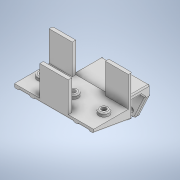
# Autodesk Inventor part: zMount1-2
Saved by Autodesk Inventor 2020 (Build 240168000, 168)
## iProperties
Created: 2020-01-08
Part Number: zMount1-2
Material: Generic
Document SubType Name: Modeling
Designer: PAB
Density: 1 g/cm^3
Appearance: Default
Author: PAB
Autodesk Inventor part; units mm, degrees
ref_plane "YZ Plane" through (0, 0, 0) normal (1, 0, 0) x (0, 1, 0)
ref_plane "XZ Plane" through (0, 0, 0) normal (0, 1, 0) x (-1, 0, 0)
ref_plane "XY Plane" through (0, 0, 0) normal (0, 0, 1) x (1, 0, 0)
sketch "Sketch1" plane through (0, 0, 0) normal (0, 1, 0) x (-1, 0, 0)
  line L0 (20.5, 16.2) -> (-20.5, 16.2)
  line L1 (-20.5, 16.2) -> (-20.5, -16.2)
  line L2 (-20.5, -16.2) -> (20.5, -16.2)
  line L3 (20.5, -16.2) -> (20.5, 16.2)
  point P0 (0, 0)
  dimension "d0" = 41
  dimension "d1" = 32.4
  constraints: 8 end point, 2 parallel, 1 horizontal, 1 perpendicular
  measures "d0" distance of L2.end L1.end
  measures "d1" distance of L1.end L0.end
extrude "Extrusion1" add sketch "Sketch1" along normal blind 3
sketch "Sketch3" plane through (0, 3, 0) normal (0, 1, 0) x (1, 0, 0)
  line L0 (-20.5, -16.2) -> (20.5, -16.2) projected
  line L1 (-20.5, 16.2) -> (-20.5, -16.2) projected
  line L2 (20.5, -16.2) -> (-20.5, -16.2)
  line L3 (-20.5, -16.2) -> (-20.5, -13.2)
  line L4 (-20.5, -13.2) -> (20.5, -13.2)
  line L5 (20.5, -13.2) -> (20.5, -16.2)
  line L6 (20.5, 16.2) -> (-20.5, 16.2) projected
  line L7 (20.5, 16.2) -> (-20.5, 16.2)
  line L8 (-20.5, 16.2) -> (-20.5, 13.2)
  line L9 (-20.5, 13.2) -> (20.5, 13.2)
  line L10 (20.5, 13.2) -> (20.5, 16.2)
  point P0 (0, 0)
  dimension "d8" = 3
  dimension "d9" = 3
  constraints: 16 end point, 4 parallel, 2 horizontal, 2 perpendicular, 2 point on line
  measures "d8" distance of L2.end L3.end
  measures "d9" distance of L8.end L7.end
extrude "Extrusion3" add sketch "Sketch3" along normal blind 25.4
sketch "Sketch4" plane through (20.5, 0, -16.2) normal (0, 0, -1) x (-1, 0, 0)
  line L0 (41, 3) -> (0, 3) projected
  line L1 (0, 28.4) -> (41, 28.4) projected
  line L2 (0, 3) -> (21.5, 3)
  line L3 (21.5, 3) -> (21.5, 28.4)
  line L4 (21.5, 28.4) -> (0, 28.4)
  line L5 (0, 28.4) -> (0, 3)
  point P0 (20.5, 0)
  dimension "d12" = 21.5
  constraints: 8 end point, 2 parallel, 1 horizontal, 1 perpendicular, 1 point on line
  measures "d12" distance of L4.end L3.end
extrude "Extrusion4" cut sketch "Sketch4" against normal blind 3
sketch "Sketch5" plane through (-20.5, 0, 16.2) normal (0, 0, 1) x (1, 0, 0)
  line L0 (41, 28.4) -> (0, 28.4) projected
  line L1 (19.5, 3) -> (41, 3) projected
  line L2 (0, 28.4) -> (21.5, 28.4)
  line L3 (21.5, 28.4) -> (21.5, 3)
  line L4 (21.5, 3) -> (0, 3)
  line L5 (0, 3) -> (0, 28.4)
  point P0 (20.5, 0)
  dimension "d15" = 21.5
  constraints: 8 end point, 2 parallel, 1 horizontal, 1 perpendicular, 1 point on line
  measures "d15" distance of L3.end L4.end
extrude "Extrusion5" cut sketch "Sketch5" against normal blind 3
sketch "Sketch6" plane through (0, 3, 0) normal (0, 1, 0) x (1, 0, 0)
  circle A0 centre (13, 0) radius 4.25
  circle A1 centre (-13, 0) radius 4.25
  line L0 (-20.5, 13.2) -> (-20.5, -16.2) projected
  line L1 (20.5, -13.2) -> (20.5, 16.2) projected
  point P0 (0, 0)
  dimension "d20" = 8.5
  dimension "d21" = 8.5
  dimension "d32" = 26
  dimension "d33" = 7.5
  dimension "d34" = 7.5
  constraints: 2 centre point
  measures "d20" diameter of A0
  measures "d21" diameter of A1
  measures "d32" distance of A0.centre A1.centre
  measures "d33" distance from line of L0 A1.centre
  measures "d34" distance from line of L1 A0.centre
extrude "Extrusion6" add sketch "Sketch6" along normal blind 3
sketch "Sketch9" plane through (20.5, 0, 16.2) normal (1, 0, 0) x (0, 0, -1)
  line L0 (32.4, 0) -> (32.4, 3) projected
  line L1 (32.4, 3) -> (0, 3)
  line L2 (0, 3) -> (0, 0)
  line L3 (0, 0) -> (32.4, 0)
  line L4 (32.4, 0) -> (32.4, 3)
  point P0 (16.2, 0)
  constraints: 8 end point, 2 parallel, 1 horizontal, 1 perpendicular
extrude "Extrusion9" add sketch "Sketch9" along normal blind 26
sketch "Sketch10" plane through (0, 3, 0) normal (0, 1, 0) x (1, 0, 0)
  circle A0 centre (39, 0) radius 4.25
  point P0 (0, 0)
  dimension "d37" = 8.5
  constraints: 1 centre point
  measures "d37" diameter of A0
extrude "Extrusion10" add sketch "Sketch10" along normal blind 3
sketch "Sketch11" plane through (0, 3, 0) normal (0, 1, 0) x (1, 0, 0)
  line L0 (46.5, 16.2) -> (46.5, -16.2) projected
  line L1 (46.5, 16.2) -> (27, 16.2)
  line L2 (27, 16.2) -> (27, 13.2)
  line L3 (27, 13.2) -> (46.5, 13.2)
  line L4 (46.5, 13.2) -> (46.5, 16.2)
  point P0 (0, 0)
  dimension "d40" = 19.5
  dimension "d41" = 3
  constraints: 8 end point, 2 parallel, 1 horizontal, 1 perpendicular
  measures "d40" distance of L3.end L2.end
  measures "d41" distance of L2.end L1.end
extrude "Extrusion11" add sketch "Sketch11" along normal blind 25.4
sketch "Sketch14" plane through (20.5, 3, 13.2) normal (1, 0, 0) x (0, 0, -1)
  line L0 (0, 0) -> (0, 25.4) projected
  line L1 (-3, 0) -> (-3, 25.4) projected
  line L2 (0, 25.4) -> (-3, 25.4)
  line L3 (-3, 25.4) -> (-3, 0)
  line L4 (-3, 0) -> (0, 0)
  line L5 (0, 0) -> (0, 25.4)
  point P0 (13.2, -3)
  constraints: 8 end point, 2 parallel, 1 horizontal, 1 perpendicular
extrude "Extrusion14" add sketch "Sketch14" along normal blind 4.5
fillet "Fillet1" radius 1 3 edges at (-17.25, 6, 0) (8.75, 6, 0) (34.75, 6, 0)
sketch "Sketch15" plane through (0, 0, 0) normal (0, -1, 0) x (1, 0, 0)
  circle A0 centre (39, 0) radius 4.25 projected
  circle A1 centre (39, 0) radius 2
  circle A2 centre (13, 0) radius 3.25 projected
  circle A3 centre (13, 0) radius 2
  circle A4 centre (-13, 0) radius 3.25 projected
  circle A5 centre (-13, 0) radius 2
  point P0 (0, 0)
  dimension "d54" = 4
  dimension "d55" = 4
  dimension "d56" = 4
  constraints: 3 centre point, 3 coincident
  measures "d54" diameter of A1
  measures "d55" diameter of A3
  measures "d56" diameter of A5
extrude "Extrusion15" cut sketch "Sketch15" against normal blind 10 contours A1 | A3 | A5
sketch "Sketch16" plane through (0, 0, 0) normal (0, -1, 0) x (1, 0, 0)
  circle A0 centre (39, 0) radius 2 projected
  circle A1 centre (39, 0) radius 3
  circle A2 centre (13, 0) radius 2 projected
  circle A3 centre (13, 0) radius 3
  circle A4 centre (-13, 0) radius 2 projected
  circle A5 centre (-13, 0) radius 3
  point P0 (0, 0)
  dimension "d59" = 6
  dimension "d60" = 6
  dimension "d61" = 6
  constraints: 3 centre point, 3 coincident
  measures "d59" diameter of A1
  measures "d60" diameter of A3
  measures "d61" diameter of A5
extrude "Extrusion16" cut sketch "Sketch16" against normal blind 3 contours A0 | A1 | A2 | A3 | A4 | A5
sketch "Sketch17" plane through (0, 0, 0) normal (0, -1, 0) x (1, 0, 0)
  line L0 (-20.5, -16.2) -> (46.5, -16.2) projected
  line L1 (46.5, -16.2) -> (-20.5, -16.2)
  line L2 (-20.5, -16.2) -> (-20.5, -12.2)
  line L3 (-20.5, -12.2) -> (46.5, -12.2)
  line L4 (46.5, -12.2) -> (46.5, -16.2)
  line L5 (-20.5, 16.2) -> (46.5, 16.2) projected
  line L6 (46.5, -12.2) -> (42.5, -12.2)
  line L7 (42.5, -12.2) -> (42.5, 16.2)
  line L8 (42.5, 16.2) -> (46.5, 16.2)
  line L9 (46.5, 16.2) -> (46.5, -12.2)
  line L10 (1, 16.2) -> (-20.5, 16.2) projected
  line L11 (-20.5, -12.2) -> (-16.5, -12.2)
  line L12 (-16.5, -12.2) -> (-16.5, 16.2)
  line L13 (-16.5, 16.2) -> (-20.5, 16.2)
  line L14 (-20.5, 16.2) -> (-20.5, -12.2)
  point P0 (0, 0)
  dimension "d64" = 4
  dimension "d65" = 4
  dimension "d66" = 4
  constraints: 24 end point, 6 parallel, 3 horizontal, 3 perpendicular, 2 point on line
  measures "d64" distance of L1.end L2.end
  measures "d65" distance of L7.end L8.end
  measures "d66" distance of L13.end L12.end
extrude "Extrusion17" add sketch "Sketch17" along normal blind 5 contours L2 L3 L4 L0 | L14 L5 L12 L3 | L3 L7 L5 L9
sketch "Sketch18" plane through (-1, 28.4, -16.2) normal (0, 0, -1) x (-1, 0, 0)
  line L0 (19.5, -33.4) -> (-47.5, -33.4) projected
  line L1 (-34.5, -33.4) -> (6.5, -33.4)
  line L2 (6.5, -33.4) -> (6.5, -29.4)
  line L3 (6.5, -29.4) -> (-34.5, -29.4)
  line L4 (-34.5, -29.4) -> (-34.5, -33.4)
  line L5 (-47.5, 0) -> (-47.5, -33.4) projected
  point P0 (-1, -28.4)
  dimension "d69" = 41
  dimension "d70" = 4
  dimension "d71" = 13
  constraints: 8 end point, 2 parallel, 1 horizontal, 1 perpendicular, 1 point on line
  measures "d69" distance of L3.end L2.end
  measures "d70" distance of L2.end L1.end
  measures "d71" distance between parallel lines of L5 L4
extrude "Extrusion18" add sketch "Sketch18" along normal blind 28.4
sketch "Sketch19" plane through (0, 0, 0) normal (0, -1, 0) x (1, 0, 0)
  line L0 (42.5, -12.2) -> (-16.5, -12.2) projected
  line L1 (-16.5, 16.2) -> (42.5, 16.2) projected
  line L2 (33.5, -12.2) -> (29.5, -12.2)
  line L3 (29.5, -12.2) -> (29.5, 16.2)
  line L4 (29.5, 16.2) -> (33.5, 16.2)
  line L5 (33.5, 16.2) -> (33.5, -12.2)
  line L6 (-7.5, -12.2) -> (-3.5, -12.2)
  line L7 (-3.5, -12.2) -> (-3.5, 16.2)
  line L8 (-3.5, 16.2) -> (-7.5, 16.2)
  line L9 (-7.5, 16.2) -> (-7.5, -12.2)
  point P0 (0, 0)
  dimension "d74" = 4
  dimension "d75" = 4
  constraints: 16 end point, 4 parallel, 4 point on line, 2 horizontal, 2 perpendicular
  measures "d74" distance of L3.end L4.end
  measures "d75" distance of L8.end L7.end
extrude "Extrusion19" add sketch "Sketch19" along normal blind 5 contours L0 L3 L1 L5 | L0 L9 L1 L7
sketch "Sketch20" plane through (0, -5, 0) normal (0, -1, 0) x (1, 0, 0)
  line L0 (-7.5, -44.6) -> (33.5, -44.6) projected
  line L1 (-7.5, -16.2) -> (-7.5, -44.6) projected
  line L2 (33.5, -44.6) -> (-7.5, -44.6)
  line L3 (-7.5, -44.6) -> (-7.5, -40.6)
  line L4 (-7.5, -40.6) -> (33.5, -40.6)
  line L5 (33.5, -40.6) -> (33.5, -44.6)
  point P0 (0, 0)
  dimension "d78" = 4
  constraints: 8 end point, 2 parallel, 1 horizontal, 1 perpendicular, 1 point on line
  measures "d78" distance of L2.end L3.end
extrude "Extrusion20" add sketch "Sketch20" along normal blind 23.8
sketch "Sketch21" plane through (0, -5, 0) normal (0, -1, 0) x (1, 0, 0)
  line L0 (-7.5, -40.6) -> (33.5, -40.6) projected
  line L1 (33.5, -40.6) -> (29.5, -40.6)
  line L2 (29.5, -40.6) -> (29.5, -36.6)
  line L3 (29.5, -36.6) -> (33.5, -36.6)
  line L4 (33.5, -36.6) -> (33.5, -40.6)
  line L5 (-7.5, -40.6) -> (-3.5, -40.6)
  line L6 (-3.5, -40.6) -> (-3.5, -36.6)
  line L7 (-3.5, -36.6) -> (-7.5, -36.6)
  line L8 (-7.5, -36.6) -> (-7.5, -40.6)
  point P0 (0, 0)
  dimension "d81" = 4
  dimension "d82" = 4
  dimension "d83" = 4
  dimension "d84" = 4
  constraints: 16 end point, 4 parallel, 2 horizontal, 2 perpendicular
  measures "d81" distance of L2.end L3.end
  measures "d82" distance of L1.end L2.end
  measures "d83" distance of L7.end L6.end
  measures "d84" distance of L6.end L5.end
extrude "Extrusion21" add sketch "Sketch21" along normal blind 4
sketch "Sketch22" plane through (-1, 28.4, -44.6) normal (0, 0, -1) x (-1, 0, 0)
  line L0 (-8.5, -57.2) -> (-19.5, -57.2)
  line L1 (-19.5, -57.2) -> (-19.5, -43.2)
  line L2 (-19.5, -43.2) -> (-8.5, -43.2)
  line L3 (-8.5, -43.2) -> (-8.5, -57.2)
  circle A0 centre (-5.5, -51.7) radius 2
  circle A1 centre (-22.5, -51.7) radius 2
  line L4 (-34.5, -37.4) -> (-30.5, -37.4) projected
  line L5 (-34.5, -37.4) -> (-25.2671, -57.2)
  line L6 (-34.5, -57.2) -> (6.5, -57.2) projected
  line L7 (-34.5, -37.4) -> (-12.6531, -37.4) construction
  line L8 (-25.2671, -57.2) -> (-34.5, -57.2)
  line L9 (-34.5, -57.2) -> (-34.5, -37.4)
  line L10 (2.5, -37.4) -> (6.5, -37.4) projected
  line L11 (6.5, -37.4) -> (-2.7329, -57.2)
  line L12 (6.5, -37.4) -> (28.3469, -37.4) construction
  line L13 (-2.7329, -57.2) -> (6.5, -57.2)
  line L14 (6.5, -37.4) -> (6.5, -57.2) projected
  line L15 (6.5, -57.2) -> (6.5, -37.4)
  point P0 (-1, -28.4)
  dimension "d87" = 11
  dimension "d88" = 14
  dimension "d89" = 4
  dimension "d90" = 4
  dimension "d91" = 65
  dimension "d92" = 115
  constraints: 24 end point, 5 horizontal, 3 perpendicular, 2 centre point, 2 equal length, 2 parallel, 2 point on line
  measures "d87" distance of L1.end L2.end
  measures "d88" distance of L0.end L1.end
  measures "d89" diameter of A0
  measures "d90" diameter of A1
  measures "d91" angle of L5 L7
  measures "d92" angle of L11 L12
extrude "Extrusion22" cut sketch "Sketch22" against normal blind 4
sketch "Sketch23" plane through (46.5, 0, 16.2) normal (1, 0, 0) x (0, 0, -1)
  line L0 (56.8, -9) -> (56.8, -5) projected
  line L1 (52.8, -5) -> (52.8, -9) projected
  line L2 (56.8, -9) -> (52.8, -5)
  line L3 (52.8, -5) -> (52.8, -9)
  line L4 (56.8, -28.8) -> (56.8, -9) projected
  line L5 (52.8, -9) -> (56.8, -9)
  line L6 (28.4, 0) -> (28.4, -5) projected
  line L7 (28.4, -5) -> (0, 0)
  line L8 (0, -5) -> (0, 3) projected
  line L9 (28.4, -5) -> (0, -5) projected
  line L10 (0, -5) -> (28.4, -5)
  point P0 (16.2, 0)
  constraints: 10 end point, 1 collinear, 1 horizontal, 1 perpendicular, 1 point on line
extrude "Extrusion23" cut sketch "Sketch23" against normal blind 67
fillet "Fillet3" radius 3 6 edges at (24.2671, -28.8, -42.6) (18.5, -28.8, -42.6) (18.5, -14.8, -42.6) (7.5, -14.8, -42.6) (7.5, -28.8, -42.6) (1.7329, -28.8, -42.6)
fillet "Fillet4" radius 1 47 edges at (2.0322, -28.3302, -44.6) (4.0721, -28.8, -44.6) (6.6213, -27.9213, -44.6) (7.5, -21.8, -44.6) (8.3787, -15.6787, -44.6) (13, -14.8, -44.6) (17.6213, -15.6787, -44.6) (18.5, -21.8, -44.6) (19.3787, -27.9213, -44.6) (21.9279, -28.8, -44.6) (23.9678, -28.3302, -44.6) (29.2874, -18.0339, -44.6) (-3.2874, -18.0339, -44.6) (2.0322, -28.3302, -40.6) (4.0721, -28.8, -40.6) (6.6213, -27.9213, -40.6) (7.5, -21.8, -40.6) (8.3787, -15.6787, -40.6) (13, -14.8, -40.6) (17.6213, -15.6787, -40.6) (18.5, -21.8, -40.6) (19.3787, -27.9213, -40.6) (21.9279, -28.8, -40.6) (23.9678, -28.3302, -40.6) (29.2874, -18.0339, -40.6) (-3.2874, -18.0339, -40.6) (-7.5, -5, -26.4) (33.5, -5, -26.4) (-7.5, -1, -30.4) (33.5, -1, -30.4) (40, -5, -16.2) (-14, -5, -16.2) (-20.5, -2.5, 2) (-16.5, -2.5, 2) (-7.5, -2.5, 2) (-3.5, -2.5, 2) (29.5, -2.5, 2) (33.5, -2.5, 2) (42.5, -2.5, 2) (46.5, -2.5, 2) (46.5, 11.7, -16.2) (-20.5, 11.7, -16.2) (13, -1, -44.6) (33.5, -5, -44.6) (-7.5, -5, -44.6) (33.5, -7, -38.6) (-7.5, -7, -38.6)
fillet "Fillet5" radius 1 6 edges at (-12, -5, -12.2) (13, -5, -12.2) (38, -5, -12.2) (38, 0, 16.2) (13, 0, 16.2) (-12, 0, 16.2)
body "Solid1"
